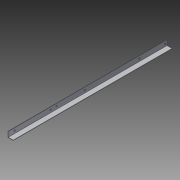
# Autodesk Inventor part: Electrical Board 1 Bracing L Channel Part 2
Saved by Autodesk Inventor 2014 SP1 (Build 180222100, 222)
## iProperties
Created: 2013-10-26
Part Number: Electrical Board 1 Bracing L Channel Part 2
Material: Aluminum 6061
Document SubType Name: Modeling
Designer: Moses
Density: 2.71 g/cm^3
Appearance: Aluminum - Flat
Mass: 31.4128 g
Surface Area: 300.75 cm^2
Volume: 11.5914 cm^3
Author: Moses
Autodesk Inventor part; units mm, degrees
ref_plane "YZ Plane" through (0, 0, 0) normal (1, 0, 0) x (0, 1, 0)
ref_plane "XZ Plane" through (0, 0, 0) normal (0, 1, 0) x (-1, 0, 0)
ref_plane "XY Plane" through (0, 0, 0) normal (0, 0, 1) x (1, 0, 0)
sketch "Sketch1" plane through (0, 0, 0) normal (0, 0, 1) x (1, 0, 0)
  line L0 (0, 0) -> (15.875, 0)
  line L1 (15.875, 0) -> (15.875, 0.7937)
  line L2 (15.875, 0.7937) -> (0.7938, 0.7937)
  line L3 (0.7938, 0.7937) -> (0.7937, 15.875)
  line L4 (0.7937, 15.875) -> (0, 15.875)
  line L5 (0, 15.875) -> (0, 0)
  dimension "d0" = 15.875
  dimension "d1" = 0.7937
  dimension "d2" = 0.7937
  constraints: 12 end point, 4 perpendicular, 2 parallel, 1 horizontal
  measures "d0" distance of L0.start L0.end
  measures "d1" distance of L0.end L1.end
  measures "d2" distance of L3.end L4.end
extrude "Extrusion1" add sketch "Sketch1" along normal blind 474.6752
sketch "Sketch2" plane through (0.7937, 0.7937, 0) normal (1, 0, 0) x (0, 0, -1)
  line L0 (0, 0) -> (0, 15.0812) projected
  line L1 (-474.6752, 0) -> (-474.6752, 15.0812) projected
  line L2 (-474.6752, 7.5406) -> (0, 7.5406) construction
  circle A0 centre (-455.6252, 112.4267) radius 2.2479 construction
  circle A1 centre (-82.55, 112.4267) radius 2.2479 construction
  circle A2 centre (-63.5127, 112.4267) radius 2.2479 construction
  circle A3 centre (-19.0627, 112.4267) radius 2.2479 construction
  circle A4 centre (-6.35, 112.4267) radius 2.2479 construction
  circle A5 centre (-246.0752, 112.4267) radius 2.2479 construction
  circle A6 centre (-347.6752, 112.4267) radius 2.2479 construction
  line L3 (0, 104.8861) -> (0, 119.9674) construction
  line L4 (0, 119.9674) -> (-474.6752, 119.9674) construction
  line L5 (-474.6752, 104.8861) -> (-474.6752, 119.9674) construction
  line L6 (0, 104.8861) -> (-474.6752, 104.8861) construction
  circle A7 centre (-455.6252, 7.5406) radius 2.2479
  circle A8 centre (-347.6752, 7.5406) radius 2.2479
  circle A9 centre (-246.0752, 7.5406) radius 2.2479
  circle A10 centre (-82.55, 7.5406) radius 2.2479
  circle A11 centre (-6.35, 7.5406) radius 2.2479
  line L7 (-455.6252, 112.4267) -> (-455.6252, 7.5406) construction
  line L8 (-347.6752, 7.5406) -> (-347.6752, 112.4267) construction
  line L9 (-246.0752, 112.4267) -> (-246.0752, 7.5406) construction
  line L10 (-82.55, 112.4267) -> (-82.55, 7.5406) construction
  line L11 (-6.35, 7.5406) -> (-6.35, 112.4267) construction
  circle A12 centre (-330.2127, 8.7312) radius 1.905 projected
  circle A13 centre (-369.6843, 112.9728) radius 1.905 projected
  point P0 (0, -0.7937)
  constraints: 12 end point, 5 centre point, 5 equal radius, 5 point on line, 3 parallel, 2 midpoint, 1 perpendicular, 1 vertical
extrude "Extrusion2" cut sketch "Sketch2" against normal through all contours A7 | A8 | A9 | A10 | A11 | A12
body "Solid1"
